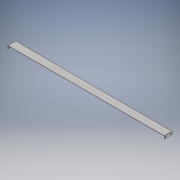
# Autodesk Inventor part: Fin
Saved by Autodesk Inventor 2017 (Build 210142000, 142)
## iProperties
Created: 2016-09-26
Part Number: Fin
Material: Stainless Steel
Document SubType Name: Sheet Metal
Designer: Andres
Density: 8 g/cm^3
Appearance: Aluminum - Polished
Sheet Metal Rule: Default_mm
Author: Andres
Autodesk Inventor part; units mm, degrees
ref_plane "YZ Plane" through (0, 0, 0) normal (1, 0, 0) x (0, 1, 0)
sketch "Sketch1" plane through (0, 0, 0) normal (0, 0, 1) x (1, 0, 0)
  line L0 (-300, 0) -> (300, 0)
  line L1 (-300, -0.76) -> (300, -0.76)
  line L2 (-300, -0.76) -> (-300, -10.76)
  line L3 (-300, -10.76) -> (-300.76, -10.76)
  line L4 (-300.76, -10.76) -> (-300.76, 0)
  line L5 (-300.76, 0) -> (-300, 0)
  line L6 (300, -0.76) -> (300, -10.76)
  line L7 (300, -10.76) -> (300.76, -10.76)
  line L8 (300.76, -10.76) -> (300.76, 0)
  line L9 (300.76, 0) -> (300, 0)
  point P0 (0, 0)
  point P1 (0, 0)
  dimension "d0" = 600
  dimension "d2" = 0.76
  dimension "d3" = 10
  dimension "d4" = 0.76
  dimension "d5" = 300
  dimension "d6" = 600
  dimension "d7" = 10
  dimension "d8" = 0.76
  constraints: 20 end point, 4 perpendicular, 3 vertical, 2 coincident, 2 horizontal, 1 midpoint, 1 parallel
  measures "d0" distance of L0.start L0.end
  measures "d2" distance between parallel lines of L0 L1
  measures "d3" distance of L1.start L2.end
  measures "d4" distance of L2.end L3.end
  measures "d5" distance from line of point (0, 0) L2
  measures "d6" distance from line of L1.end L2
  measures "d7" distance of L1.end L6.end
  measures "d8" distance of L6.end L7.end
extrude "Extrusion1" add sketch "Sketch1" along normal blind 30
fillet "Fillet1" radius 1 1 edges at (-300.76, 0, 15)
fillet "Fillet2" radius 1 1 edges at (300.76, 0, 15)
ref_plane "Work Plane1" through (300.76, -10.76, 30) normal (1, 0, 0) x (0, 0, -1)
sketch "Sketch2" plane through (300.76, -10.76, 30) normal (1, 0, 0) x (0, 0, -1)
  line L0 (0, 9.76) -> (30, 9.76) projected
  line L1 (0, 0) -> (0, 9.76) projected
  line L2 (30, 0) -> (0, 0) projected
  line L3 (30, 9.76) -> (30, 0) projected
  point P0 (30, 10.76)
  point P1 (5, 5)
  point P2 (25, 5)
  dimension "d14" = 5
  dimension "d15" = 5
  dimension "d16" = 5
  dimension "d17" = 5
  measures "d14" distance from line of L2 point (25, 5)
  measures "d15" distance from line of L3 point (25, 5)
  measures "d16" distance from line of L2 point (5, 5)
  measures "d17" distance from line of L1 point (5, 5)
hole "Hole1" at (300.76, -5.76, 25) at (300.76, -5.76, 5) direction (-1, 0, 0) diameter 4 depth 0.76 tip angle 118
ref_plane "Work Plane2" through (-300.76, -10.76, 0) normal (-1, 0, 0) x (0, 0, 1)
sketch "Sketch3" plane through (-300.76, -10.76, 0) normal (-1, 0, 0) x (0, 0, 1)
  line L0 (0, 0) -> (30, 0) projected
  line L1 (0, 0) -> (0, 9.76) projected
  line L2 (30, 9.76) -> (30, 0) projected
  point P0 (0, 10.76)
  point P1 (5, 5)
  point P2 (25, 5)
  dimension "d26" = 5
  dimension "d27" = 5
  dimension "d28" = 5
  dimension "d29" = 5
  measures "d26" distance from line of L0 point (5, 5)
  measures "d27" distance from line of point (5, 5) L1
  measures "d28" distance from line of L2 point (25, 5)
  measures "d29" distance from line of L0 point (25, 5)
hole "Hole2" at (-300.76, -5.76, 5) at (-300.76, -5.76, 25) direction (1, 0, 0) diameter 4 depth 0.76 tip angle 118
equation "\"BendRadius\" = Thickness"
equation "\"BendReliefWidth\" = Thickness"
equation "\"BendReliefDepth\" = 0.5 * Thickness"
equation "\"CornerReliefSize\" = 4 * Thickness"
equation "\"MinimumRemnant\" = 2 * Thickness"
equation "\"TransitionRadius\" = BendRadius"
equation "\"JacobiRadiusSize\" = BendRadius"
equation "\"GapSize\" = Thickness"
equation "\"Thickness\" = 0.76"
body "Solid1"
